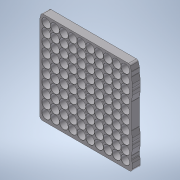
# Autodesk Inventor part: J008197
Saved by Autodesk Inventor 2020.3 (Build 243373000, 373)
## iProperties
RuleStatus: InUse
AfterDocSave0: file://Part Number Cleaner
Created: 2018-09-09
Material: ALUMINUM, 6061-T651
Vendor: HHMI: JRC - ID&F
Document SubType Name: Modeling
Designer: arnoldj
Density: 2.7 g/cm^3
Appearance: Metal-AL-6061 (Machined)
Part Number: J008197
Project: COMMON
Description: VIAL PRESS CAP TRAY UPPER
LAB/DEPT: FLY FACILITY (SHARED RESOURCE)
REQUESTING SCIENTIST: LAVERTY, TODD
SURFACE ROUGHNESS: 63 Ra
DESIGN DEPARTMENT: HHMI: JRC - ID&F
SPECIAL FINISH: NONE
ALTERED ITEM PART NUMBER: N/A
ALTERED ITEM VENDOR: N/A
ALTERED ITEM DESCRIPTION: N/A
Author: arnoldj
Revision Number: A
Autodesk Inventor part; units mm, degrees
ref_plane "YZ Plane" through (0, 0, 0) normal (1, 0, 0) x (0, 1, 0)
ref_plane "XZ Plane" through (0, 0, 0) normal (0, 1, 0) x (-1, 0, 0)
sketch "Sketch1" plane through (0, 0, 0) normal (0, 0, 1) x (1, 0, 0)
  line L0 (0, 210.312) -> (0, -212.852) projected
  line L1 (-210.312, 0) -> (212.852, 0) projected
  line L2 (149.86, -152.4) -> (-149.86, -152.4)
  line L3 (-149.86, -152.4) -> (-149.86, 149.86)
  line L4 (-149.86, 149.86) -> (149.86, 149.86)
  line L5 (149.86, 149.86) -> (149.86, -152.4)
  line L6 (129.159, -129.159) -> (-129.159, -129.159)
  line L7 (-129.159, -129.159) -> (-129.159, 129.159)
  line L8 (-129.159, 129.159) -> (129.159, 129.159)
  line L9 (129.159, 129.159) -> (129.159, -129.159)
  line L10 (129.159, -129.159) -> (-129.159, 129.159) construction
  line L11 (-129.159, -129.159) -> (129.159, 129.159) construction
  line L12 (76.2, -76.2) -> (-76.2, -76.2) construction
  line L13 (-76.2, -76.2) -> (-76.2, 76.2) construction
  line L14 (-76.2, 76.2) -> (76.2, 76.2) construction
  line L15 (76.2, 76.2) -> (76.2, -76.2) construction
  line L16 (76.2, -76.2) -> (-76.2, 76.2) construction
  line L17 (-76.2, -76.2) -> (76.2, 76.2) construction
  line L18 (114.808, -114.808) -> (-114.808, -114.808) construction
  line L19 (-114.808, -114.808) -> (-114.808, 114.808) construction
  line L20 (-114.808, 114.808) -> (114.808, 114.808) construction
  line L21 (114.808, 114.808) -> (114.808, -114.808) construction
  line L22 (114.808, -114.808) -> (-114.808, 114.808) construction
  line L23 (-114.808, -114.808) -> (114.808, 114.808) construction
  line L24 (146.05, -146.05) -> (-146.05, -146.05) construction
  line L25 (-146.05, -146.05) -> (-146.05, 146.05) construction
  line L26 (-146.05, 146.05) -> (146.05, 146.05) construction
  line L27 (146.05, 146.05) -> (146.05, -146.05) construction
  line L28 (152.4, 65.405) -> (149.86, 65.405)
  line L29 (149.86, 65.405) -> (149.86, 97.155)
  line L30 (149.86, 97.155) -> (152.4, 97.155)
  line L31 (152.4, 65.405) -> (149.86, 97.155) construction
  line L32 (149.86, 65.405) -> (152.4, 97.155) construction
  line L33 (152.4, 97.155) -> (149.86, 116.4482)
  line L34 (152.4, 65.405) -> (149.86, 46.1118)
  line L35 (149.86, -152.4) -> (152.4, -152.4)
  line L36 (152.4, -152.4) -> (152.4, -127)
  line L37 (152.4, -127) -> (149.86, -127)
  line L38 (149.86, -127) -> (149.86, -152.4)
  line L39 (152.4, -127) -> (149.86, -117.5206)
  line L40 (152.4, 97.155) -> (152.4, 65.405)
  point P0 (0, 0)
  point P1 (151.13, 81.28)
  point P2 (151.13, 81.28)
  dimension "d0" = 129.159
  dimension "d1" = 129.159
  dimension "d23" = 152.4
  dimension "d36" = 114.808
  dimension "d63" = 292.1
  dimension "d89" = 31.75
  dimension "d91" = 81.28
  dimension "d105" = 52.705
  dimension "d135" = 149.86
  dimension "d136" = 149.86
  dimension "d138" = 152.4
  dimension "d146" = 149.86
  dimension "d148" = 7.5
  dimension "d149" = 7.5
  dimension "d159" = 2.54
  dimension "d160" = 25.4
  dimension "d161" = 15
  dimension "d165" = 2.54
  constraints: 78 end point, 13 parallel, 9 midpoint, 7 horizontal, 7 perpendicular, 5 coincident, 5 point on line, 1 vertical
  measures "d0" distance from line of L0 L7.end
  measures "d1" distance from line of L1 L7.end
  measures "d23" distance of L13.end L14.end
  measures "d36" distance from line of L0 L19.end
  measures "d63" distance of L25.end L26.end
  measures "d89" distance of L30.end L28.start
  measures "d91" distance from line of L1 point (151.13, 81.28)
  measures "d105" distance from line of L29.end L4
  measures "d135" distance between parallel lines of L0 L3
  measures "d136" distance between parallel lines of L1 L4
  measures "d138" distance between parallel lines of L1 L2
  measures "d146" distance between parallel lines of L0 L5
  measures "d148" angle of L33 L5
  measures "d149" angle of L34 L5
  measures "d159" distance of L2.start L35.end
  measures "d160" distance of L35.end L36.end
  measures "d161" angle of L5 L39
  measures "d165" distance of L28.start L28.end
extrude "Extrusion1" add sketch "Sketch1" against normal blind 25.908 contours L4 L5 L1 L9 L8 L0 | L0 L8 L7 L1 L3 L4 | L8 L9 L1 L0 | L0 L1 L7 L8 | L1 L9 L6 L0 | L0 L6 L7 L1 | L1 L7 L6 L0 L2 L3 | L6 L9 L1 L5 L2 L0
hole "Hole1" at (-129.159, 129.159, 0) direction (0, 0, -1) diameter 28.067 end through all countersink diameter 29.1084 countersink angle 82
sketch "Sketch15" plane through (0, 0, -25.908) normal (0, 0, -1) x (-1, 0, 0)
  point P0 (0, 0)
  point P1 (114.808, 114.808)
hole "Hole7" at (-114.808, 114.808, -25.908) direction (0, 0, 1) diameter 3.2512 end through all
pattern_linear "Rectangular Pattern1" count 10 spacing 28.702 along (1, 0, 0) count 10 spacing 28.702 along (0, -1, 0) of "Hole1"
pattern_linear "Rectangular Pattern6" count 5 spacing 57.404 along (1, 0, 0) count 5 spacing 57.404 along (0, -1, 0) of "Hole7"
extrude "Extrusion8" add sketch "Sketch1" against normal up to surface (25.908 mm away) contours L33 L30 L5 | L30 L40 L28 L5 | L28 L34 L5
sketch "Sketch11" plane through (0, 0, 0) normal (0, 0, 1) x (1, 0, 0)
  line L0 (152.4, 97.155) -> (152.4, 65.405) projected
  circle A0 centre (165.989, 81.28) radius 14.4272
  line L1 (149.86, 149.86) -> (149.86, -152.4) projected
  point P0 (0, 0)
  point P1 (151.13, 81.28)
  dimension "d170" = 28.8544
  dimension "d171" = 16.129
  constraints: 1 centre point, 1 horizontal alignment
  measures "d170" diameter of A0
  measures "d171" distance from line of A0.centre L1
extrude "Extrusion11" cut sketch "Sketch11" against normal through all
fillet "Fillet9" radius 12.7 2 edges at (149.86, 116.4482, -12.954) (149.86, 46.1118, -12.954)
fillet "Fillet2" radius 9.525 1 edges at (-149.86, -152.4, -12.954)
chamfer "Chamfer7" distance 19.05 angle 15 1 edges at (149.86, 149.86, -12.954) measured on face at (149.86, 139.0002, -17.272)
chamfer "Chamfer9" distance 19.05 angle 15 1 edges at (-149.86, 149.86, -12.954) measured on face at (-149.86, -45.2967, -8.636)
fillet "Fillet5" radius 6.35 4 edges at (144.7556, 149.86, -12.954) (149.86, 130.81, -12.954) (-144.7556, 149.86, -12.954) (-149.86, 130.81, -12.954)
pattern_linear "Rectangular Pattern4" count 2 spacing 152.4 along (0, -1, 0) of "Fillet9", "Extrusion8", "Extrusion11"
extrude "Extrusion9" add sketch "Sketch1" against normal up to surface (25.908 mm away) contours L28 L34 L5 | L5 L37 L36 L35 | L39 L37 L5
fillet "Fillet10" radius 12.7 1 edges at (149.86, -117.5206, -12.954)
ref_plane "Work Plane1" through (0, 0, -8.636) normal (0, 0, -1) x (-1, 0, 0)
sketch "Sketch5" plane through (0, 0, 0) normal (0, 0, 1) x (1, 0, 0)
  line L0 (0, 210.312) -> (0, -212.852) projected
  line L1 (-198.374, 0) -> (207.899, 0) projected
  line L2 (51.054, -148.59) -> (121.158, -148.59) construction
  line L3 (149.86, -152.4) -> (-140.335, -152.4) construction
  line L4 (149.86, 149.86) -> (149.86, -152.4) projected
  circle A0 centre (129.159, -129.159) radius 15.875 construction
  line L5 (149.86, -143.51) -> (86.1178, -143.51) construction
  point P0 (0, 0)
  point P1 (86.106, -148.59)
  point P2 (149.86, 129.974)
  point P3 (57.404, -148.59)
  point P4 (114.808, -148.59)
  dimension "d124" = 3.81
  dimension "d126" = 31.75
  dimension "d175" = 6.35
  dimension "d177" = 86.106
  dimension "d178" = 28.702
  dimension "d179" = 28.702
  constraints: 4 end point, 3 point on line, 2 horizontal, 1 centre point, 1 coincident, 1 midpoint
  measures "d124" distance between parallel lines of L3 L2
  measures "d126" diameter of A0
  measures "d175" distance of point (114.808, -148.59) L2.end
  measures "d177" distance from line of L0 point (86.106, -148.59)
  measures "d178" distance of point (86.106, -148.59) point (57.404, -148.59)
  measures "d179" distance of point (114.808, -148.59) point (86.106, -148.59)
hole "Hole6" [suppressed]
sketch "Sketch14" plane through (0, 0, 0) normal (0, 0, 1) x (1, 0, 0)
  line L0 (149.9687, 46.9371) -> (152.4, 65.405) projected
  line L1 (152.4, 65.405) -> (152.4, 76.4341) projected
  arc A0 (152.4, 86.1259) -> (152.4, 76.4341) centre (165.989, 81.28) ccw projected
  line L2 (152.4, 86.1259) -> (152.4, 97.155) projected
  line L3 (152.4, 97.155) -> (149.9687, 115.6229) projected
  arc A1 (149.86, 117.2806) -> (149.9687, 115.6229) centre (162.56, 117.2806) ccw projected
  line L4 (149.86, 129.974) -> (149.86, 117.2806) projected
  arc A2 (149.86, 129.974) -> (149.6436, 131.6175) centre (143.51, 129.974) ccw projected
  line L5 (146.0167, 145.1535) -> (149.6436, 131.6175) projected
  arc A3 (146.0167, 145.1535) -> (139.883, 149.86) centre (139.883, 143.51) ccw projected
  line L6 (-139.883, 149.86) -> (139.883, 149.86) projected
  arc A4 (-139.883, 149.86) -> (-146.0167, 145.1535) centre (-139.883, 143.51) ccw projected
  line L7 (-149.6436, 131.6175) -> (-146.0167, 145.1535) projected
  arc A5 (-149.6436, 131.6175) -> (-149.86, 129.974) centre (-143.51, 129.974) ccw projected
  line L8 (-149.86, -142.875) -> (-149.86, 129.974) projected
  arc A6 (-149.86, -142.875) -> (-140.335, -152.4) centre (-140.335, -142.875) ccw projected
  line L9 (152.4, -152.4) -> (-140.335, -152.4) projected
  line L10 (152.4, -152.4) -> (152.4, -127) projected
  line L11 (152.4, -127) -> (150.2927, -119.1356) projected
  arc A7 (149.86, -115.8486) -> (150.2927, -119.1356) centre (162.56, -115.8486) ccw projected
  line L12 (149.86, -107.1206) -> (149.86, -115.8486) projected
  arc A8 (149.9687, -105.4629) -> (149.86, -107.1206) centre (162.56, -107.1206) ccw projected
  line L13 (149.9687, -105.4629) -> (152.4, -86.995) projected
  line L14 (152.4, -86.995) -> (152.4, -75.9659) projected
  arc A9 (152.4, -66.2741) -> (152.4, -75.9659) centre (165.989, -71.12) ccw projected
  line L15 (152.4, -66.2741) -> (152.4, -55.245) projected
  line L16 (152.4, -55.245) -> (149.9687, -36.7771) projected
  arc A10 (149.86, -35.1194) -> (149.9687, -36.7771) centre (162.56, -35.1194) ccw projected
  line L17 (149.86, 45.2794) -> (149.86, -35.1194) projected
  arc A11 (149.9687, 46.9371) -> (149.86, 45.2794) centre (162.56, 45.2794) ccw projected
  arc A12 (53.34, -145.542) -> (61.468, -145.542) centre (57.404, -148.59) ccw
  line L18 (52.324, -148.59) -> (62.484, -148.59)
  line L19 (62.484, -148.59) -> (62.484, -153.67)
  line L20 (62.484, -153.67) -> (52.324, -153.67)
  line L21 (52.324, -153.67) -> (52.324, -148.59)
  line L22 (53.34, -145.542) -> (61.468, -145.542)
  circle A13 centre (57.404, -148.59) radius 3.048 construction
  point P0 (0, 0)
  dimension "d180" = 10.16
  dimension "d230" = 6.096
  constraints: 10 end point, 3 point on circle, 3 tangent, 2 centre point, 2 horizontal, 2 parallel, 1 coincident, 1 perpendicular
  measures "d180" diameter of A12
  measures "d230" diameter of A13
extrude "Extrusion12" [suppressed]
pattern_linear "Rectangular Pattern5" [suppressed]
fillet "Fillet11" [suppressed]
sketch "Sketch16" plane through (0, 0, 0) normal (0, 0, 1) x (1, 0, 0)
  circle A0 centre (-71.755, 71.755) radius 14.0335 projected
  circle A1 centre (-71.755, 100.457) radius 14.0335 projected
  circle A2 centre (-71.755, 71.755) radius 14.0843
  circle A3 centre (-71.755, 100.457) radius 14.0843
  line L0 (-71.755, 86.3727) -> (-71.755, 85.8393)
  line L1 (-71.755, 86.4235) -> (-71.755, 85.7885)
  point P0 (0, 0)
  dimension "d201" = 28.1686
  dimension "d202" = 28.1686
  dimension "d203" = 28.067
  dimension "d205" = 0.635
  constraints: 4 end point, 4 vertical alignment, 2 coincident, 1 vertical, 6 other
  measures "d205" distance of L1.start L1.end
sketch "Sketch17" plane through (0, 0, 0) normal (0, 0, 1) x (1, 0, 0)
  circle A0 centre (-129.159, 129.159) radius 14.0335 projected
  circle A1 centre (-114.808, 114.808) radius 1.6256 projected
  circle A2 centre (-100.457, 129.159) radius 14.0335 projected
  line L0 (-143.51, 143.51) -> (-114.808, 143.51) construction
  line L1 (-114.808, 143.51) -> (-114.808, 114.808) construction
  line L2 (-114.808, 114.808) -> (-143.51, 114.808) construction
  line L3 (-143.51, 114.808) -> (-143.51, 143.51) construction
  line L4 (-143.51, 143.51) -> (-114.808, 114.808) construction
  line L5 (-114.808, 143.51) -> (-143.51, 114.808) construction
  circle A3 centre (-143.51, 143.51) radius 1.6256 construction
  circle A4 centre (57.404, -114.808) radius 1.6256 construction
  circle A5 centre (71.755, -129.159) radius 14.0335 construction
  line L6 (86.106, -143.51) -> (57.404, -143.51) construction
  line L7 (57.404, -143.51) -> (57.404, -114.808) construction
  line L8 (57.404, -114.808) -> (86.106, -114.808) construction
  line L9 (86.106, -114.808) -> (86.106, -143.51) construction
  line L10 (86.106, -143.51) -> (57.404, -114.808) construction
  line L11 (57.404, -143.51) -> (86.106, -114.808) construction
  circle A6 centre (114.808, -114.808) radius 1.6256 construction
  circle A7 centre (129.159, -129.159) radius 14.0335 construction
  line L12 (143.51, -143.51) -> (114.808, -143.51) construction
  line L13 (114.808, -143.51) -> (114.808, -114.808) construction
  line L14 (114.808, -114.808) -> (143.51, -114.808) construction
  line L15 (143.51, -114.808) -> (143.51, -143.51) construction
  line L16 (143.51, -143.51) -> (114.808, -114.808) construction
  line L17 (114.808, -143.51) -> (143.51, -114.808) construction
  line L18 (-149.6436, 131.6175) -> (-146.0167, 145.1535) construction
  line L19 (-145.0802, 143.9307) -> (-145.9239, 140.7822) construction
  point P0 (0, 0)
  dimension "d209" = 3.2512
  dimension "d206" = 14.351
  dimension "d207" = 14.351
  dimension "d208" = 3.2512
  dimension "d210" = 1.221
  constraints: 38 end point, 7 parallel, 6 midpoint, 3 horizontal, 3 perpendicular, 2 coincident, 4 other
  measures "d206" horizontal distance of A0.centre L1.end
  measures "d207" horizontal distance of A0.centre L1.end
  measures "d208" diameter of A6
  measures "d210" distance between parallel lines of L19 L18
hole "Hole8" [suppressed]
pattern_linear "Rectangular Pattern7" [suppressed]
pattern_linear "Rectangular Pattern8" [suppressed]
pattern_linear "Rectangular Pattern9" [suppressed]
pattern_linear "Rectangular Pattern10" [suppressed]
fillet "Fillet12" [suppressed]
fillet "Fillet13" radius 9.525 1 edges at (152.4, -152.4, -12.954)
equation "\"d1\" = d0"
body "Solid1"
